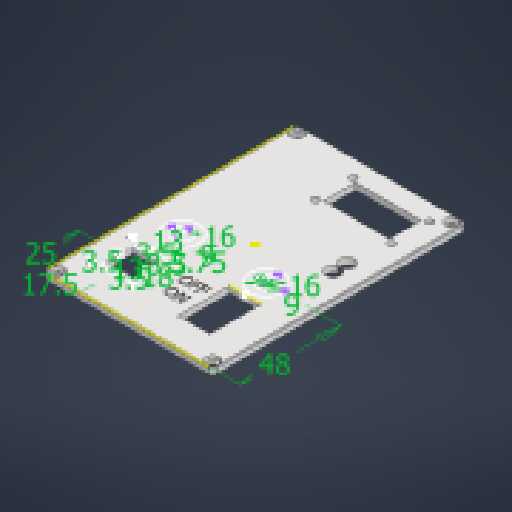
# Autodesk Inventor part: PCB_Housing_06_V4
Saved by Autodesk Inventor 2026.2 (Build 302298000, 298)
## iProperties
Created: 2026-03-17
Part Number: PCB_Housing_06_V4
Material: Generic
Document SubType Name: Modeling
Designer: vckot
Density: 1 g/cm^3
Appearance: Default
Author: vckot
Autodesk Inventor part; units mm, degrees
ref_plane "YZ Plane" through (0, 0, 0) normal (1, 0, 0) x (0, 1, 0)
ref_plane "XZ Plane" through (0, 0, 0) normal (0, 1, 0) x (-1, 0, 0)
ref_plane "XY Plane" through (0, 0, 0) normal (0, 0, 1) x (1, 0, 0)
sketch "Sketch1" plane through (0, 0, 0) normal (0, 1, 0) x (-1, 0, 0)
  line L0 (-40, 60) -> (40, 60)
  line L1 (40, 60) -> (40, -60)
  line L2 (40, -60) -> (-40, -60)
  line L3 (-40, -60) -> (-40, 60)
  line L4 (-40, 60) -> (40, -60) construction
  line L5 (40, 60) -> (-40, -60) construction
  point P0 (0, 0)
  dimension "d0" = 120
  dimension "d1" = 80
  constraints: 12 end point, 2 midpoint, 2 parallel, 1 horizontal, 1 perpendicular
  measures "d0" distance of L0.end L1.end
  measures "d1" distance of L0.start L0.end
extrude "Extrusion1" add sketch "Sketch1" along normal blind 3
sketch "Sketch2" plane through (0, 3, 0) normal (0, 1, 0) x (1, 0, 0)
  circle A0 centre (36.5, -56.5) radius 2.25 projected
  circle A1 centre (-36.5, 56.5) radius 2.25 projected
  circle A2 centre (36.5, 56.5) radius 2.25
  circle A3 centre (-36.5, -56.5) radius 2.25
  point P0 (0, 0)
  constraints: 2 centre point, 2 equal radius, 2 horizontal alignment, 2 vertical alignment
hole "Hole1" at (36.5, 3, 56.5) at (-36.5, 3, -56.5) at (36.5, 3, -56.5) at (-36.5, 3, 56.5) direction (0, -1, 0) diameter 3.75 depth 8 tip angle 118 counterbore diameter 6 counterbore depth 2
sketch "Sketch3" plane through (0, 3, 0) normal (0, 1, 0) x (1, 0, 0)
  line L0 (24.241, -45.543499) -> (24.241, -22.556499)
  line L1 (10.779, -45.543499) -> (24.241, -45.543499)
  line L2 (10.779, -22.556499) -> (10.779, -45.543499)
  line L3 (10.779, -22.556499) -> (24.241, -22.556499)
  arc A0 (26.856832, 17.449996) -> (30.143167, 17.449996) centre (28.499999, 14.999996) ccw
  arc A1 (26.856832, 10.949996) -> (30.143167, 10.949996) centre (28.499999, 8.499996) ccw
  circle A2 centre (28.499999, 8.499996) radius 2.95
  circle A3 centre (28.499999, 14.999996) radius 2.95
  line L4 (28, 35.5) -> (-2, 35.5)
  line L5 (-2, 35.5) -> (-2, 49.5)
  line L6 (-2, 49.5) -> (28, 49.5)
  line L7 (28, 49.5) -> (28, 35.5)
  circle A4 centre (-7, 34) radius 1.1
  circle A5 centre (30, 34) radius 1.1
  circle A6 centre (30, 52) radius 1.1
  circle A7 centre (-7, 52) radius 1.1
  line L8 (31.5, 32.5) -> (31.5, 53.5)
  line L9 (31.5, 53.5) -> (-8.5, 53.5)
  line L10 (-8.5, 53.5) -> (-8.5, 32.5)
  line L11 (-8.5, 32.5) -> (31.5, 32.5)
  point P0 (0, 0)
  point P1 (26.856832, 10.949996)
  constraints: 2 centre point, 2 coincident, 2 concentric, 2 end point, 1 horizontal
extrude "Extrusion2" cut sketch "Sketch3" against normal through all contours L1 L2 L3 L0 | A3 A0 | A2 A1 | L4 L5 L6 L7
sketch "Sketch5" plane through (0, 3, 0) normal (0, 1, 0) x (1, 0, 0)
  circle A0 centre (-5, 33.5) radius 1.75
  circle A1 centre (-5, 51.5) radius 1.75
  circle A2 centre (31, 51.5) radius 1.75
  circle A3 centre (31, 33.5) radius 1.75
  line L0 (28, 35.5) -> (-2, 35.5) projected
  line L1 (-2, 35.5) -> (-2, 49.5) projected
  line L2 (-2, 49.5) -> (28, 49.5) projected
  line L3 (28, 49.5) -> (28, 35.5) projected
  point P0 (0, 0)
  dimension "d27" = 3.5
  dimension "d28" = 2
  dimension "d29" = 3
  dimension "d30" = 2
  dimension "d31" = 3
  dimension "d32" = 3
  dimension "d33" = 3
  dimension "d34" = 2
  dimension "d35" = 2
  constraints: 4 centre point, 3 equal radius
  measures "d27" diameter of A0
  measures "d28" distance from line of A0.centre L0
  measures "d29" distance from line of L1 A0.centre
  measures "d30" distance from line of L2 A1.centre
  measures "d31" distance from line of L1 A1.centre
  measures "d32" distance from line of L3 A2.centre
  measures "d33" distance from line of L3 A3.centre
  measures "d34" distance from line of L0 A3.centre
  measures "d35" distance from line of L2 A2.centre
extrude "Extrusion4" cut sketch "Sketch5" against normal through all contours A0 | A1 | A2 | A3
thicken "Thicken1" operation add thickness 0.5 both sides no extend neighbours yes toward (0, 0, -1) faces at (18, 2, -49.5) (-2, 2, -44.833333) (28, 2, -40.166667) (8, 2, -35.5)
thicken "Thicken2" operation add thickness 0.5 both sides no extend neighbours yes toward (0.6830158, 0, -0.7304036) faces at (30.514896, 2, -17.154687)
thicken "Thicken3" operation add thickness 0.5 both sides no extend neighbours yes toward (0.6830158, 0, -0.7304036) faces at (30.514896, 2, -10.654687)
thicken "Thicken4" operation add thickness 0.75 both sides no extend neighbours yes toward (1, 0, 0) faces at (24.241, 1, 30.218832) (19.753666, 2, 22.556499) (10.779, 2, 30.218832) (15.266333, 2, 45.543499)
sketch "Sketch4" plane through (0, 3, 0) normal (0, 1, 0) x (1, 0, 0)
  line L0 (-9.166236, -22.743083) -> (11.364424, -22.743083) construction
  line L1 (11.364424, -22.743083) -> (11.364424, -45.356916) construction
  line L2 (11.364424, -45.356916) -> (-9.166236, -45.356916) construction
  line L3 (-9.166236, -45.356916) -> (-9.166236, -22.743083) construction
  line L4 (10.029, -21.806499) -> (24.991, -21.806499)
  line L5 (10.029, -46.293499) -> (10.029, -21.806499)
  spline S0 degree 2 poles (-0.87619, -28.005128) (-0.59256, -28.337381) (-0.276514, -29.309828) (-0.276514, -29.933815) knots 0 0 0 1 2 2 2
  spline S1 degree 2 poles (-0.276514, -29.933815) (-0.276514, -30.541595) (-0.584456, -31.526197) (-0.87619, -31.85845) knots 0 0 0 1 2 2 2
  spline S2 degree 2 poles (-0.87619, -31.85845) (-1.184132, -32.206911) (-1.998556, -32.539163) (-2.488832, -32.539163) knots 0 0 0 1 2 2 2
  spline S3 degree 2 poles (-2.488832, -32.539163) (-2.995315, -32.539163) (-3.805688, -32.194755) (-4.101474, -31.85845) knots 0 0 0 1 2 2 2
  spline S4 degree 2 poles (-4.101474, -31.85845) (-4.389156, -31.526197) (-4.697098, -30.549698) (-4.697098, -29.933815) knots 0 0 0 1 2 2 2
  spline S5 degree 2 poles (-4.697098, -29.933815) (-4.697098, -29.305776) (-4.385104, -28.349536) (-4.097422, -28.005128) knots 0 0 0 1 2 2 2
  spline S6 degree 2 poles (-4.097422, -28.005128) (-3.805688, -27.672875) (-2.991263, -27.328467) (-2.488832, -27.328467) knots 0 0 0 1 2 2 2
  spline S7 degree 2 poles (-2.488832, -27.328467) (-1.978297, -27.328467) (-1.159821, -27.685031) (-0.87619, -28.005128) knots 0 0 0 1 2 2 2
  spline S8 degree 2 poles (-0.969383, -29.933815) (-0.969383, -29.439488) (-1.184132, -28.673685) (-1.378621, -28.42247) knots 0 0 0 1 2 2 2
  spline S9 degree 2 poles (-1.378621, -28.42247) (-1.577162, -28.16315) (-2.13632, -27.903831) (-2.48478, -27.903831) knots 0 0 0 1 2 2 2
  spline S10 degree 2 poles (-2.48478, -27.903831) (-2.845396, -27.903831) (-3.388346, -28.155047) (-3.594991, -28.42247) knots 0 0 0 1 2 2 2
  spline S11 degree 2 poles (-3.594991, -28.42247) (-3.793532, -28.677737) (-4.004229, -29.447591) (-4.004229, -29.933815) knots 0 0 0 1 2 2 2
  spline S12 degree 2 poles (-4.004229, -29.933815) (-4.004229, -30.918418) (-3.177649, -31.963799) (-2.48478, -31.963799) knots 0 0 0 1 2 2 2
  spline S13 degree 2 poles (-2.48478, -31.963799) (-1.791911, -31.963799) (-0.969383, -30.918418) (-0.969383, -29.933815) knots 0 0 0 1 2 2 2
  line L6 (3.443097, -28.025387) -> (1.117327, -28.025387)
  line L7 (1.117327, -28.025387) -> (1.117327, -29.435436)
  line L8 (1.117327, -29.435436) -> (3.345852, -29.435436)
  line L9 (3.345852, -29.435436) -> (3.345852, -30.027008)
  line L10 (3.345852, -30.027008) -> (1.117327, -30.027008)
  line L11 (1.117327, -30.027008) -> (1.117327, -32.433815)
  line L12 (1.117327, -32.433815) -> (0.452821, -32.433815)
  line L13 (0.452821, -32.433815) -> (0.452821, -27.433815)
  line L14 (0.452821, -27.433815) -> (3.443097, -27.433815)
  line L15 (3.443097, -27.433815) -> (3.443097, -28.025387)
  line L16 (7.028996, -28.025387) -> (4.703226, -28.025387)
  line L17 (4.703226, -28.025387) -> (4.703226, -29.435436)
  line L18 (4.703226, -29.435436) -> (6.931752, -29.435436)
  line L19 (6.931752, -29.435436) -> (6.931752, -30.027008)
  line L20 (6.931752, -30.027008) -> (4.703226, -30.027008)
  line L21 (4.703226, -30.027008) -> (4.703226, -32.433815)
  line L22 (4.703226, -32.433815) -> (4.038721, -32.433815)
  line L23 (4.038721, -32.433815) -> (4.038721, -27.433815)
  line L24 (4.038721, -27.433815) -> (7.028996, -27.433815)
  line L25 (7.028996, -27.433815) -> (7.028996, -28.025387)
  spline S14 degree 2 poles (0.414329, -36.237496) (0.697959, -36.569749) (1.014005, -37.542196) (1.014005, -38.166183) knots 0 0 0 1 2 2 2
  spline S15 degree 2 poles (1.014005, -38.166183) (1.014005, -38.773963) (0.706063, -39.758566) (0.414329, -40.090819) knots 0 0 0 1 2 2 2
  spline S16 degree 2 poles (0.414329, -40.090819) (0.106387, -40.439279) (-0.708037, -40.771532) (-1.198313, -40.771532) knots 0 0 0 1 2 2 2
  spline S17 degree 2 poles (-1.198313, -40.771532) (-1.704796, -40.771532) (-2.515169, -40.427123) (-2.810955, -40.090819) knots 0 0 0 1 2 2 2
  spline S18 degree 2 poles (-2.810955, -40.090819) (-3.098637, -39.758566) (-3.406579, -38.782067) (-3.406579, -38.166183) knots 0 0 0 1 2 2 2
  spline S19 degree 2 poles (-3.406579, -38.166183) (-3.406579, -37.538144) (-3.094585, -36.581904) (-2.806903, -36.237496) knots 0 0 0 1 2 2 2
  spline S20 degree 2 poles (-2.806903, -36.237496) (-2.515169, -35.905243) (-1.700744, -35.560835) (-1.198313, -35.560835) knots 0 0 0 1 2 2 2
  spline S21 degree 2 poles (-1.198313, -35.560835) (-0.687778, -35.560835) (0.130698, -35.917399) (0.414329, -36.237496) knots 0 0 0 1 2 2 2
  spline S22 degree 2 poles (0.321136, -38.166183) (0.321136, -37.671856) (0.106387, -36.906054) (-0.088102, -36.654838) knots 0 0 0 1 2 2 2
  spline S23 degree 2 poles (-0.088102, -36.654838) (-0.286644, -36.395519) (-0.845801, -36.136199) (-1.194261, -36.136199) knots 0 0 0 1 2 2 2
  spline S24 degree 2 poles (-1.194261, -36.136199) (-1.554877, -36.136199) (-2.097827, -36.387415) (-2.304472, -36.654838) knots 0 0 0 1 2 2 2
  spline S25 degree 2 poles (-2.304472, -36.654838) (-2.503013, -36.910105) (-2.71371, -37.67996) (-2.71371, -38.166183) knots 0 0 0 1 2 2 2
  spline S26 degree 2 poles (-2.71371, -38.166183) (-2.71371, -39.150786) (-1.88713, -40.196167) (-1.194261, -40.196167) knots 0 0 0 1 2 2 2
  spline S27 degree 2 poles (-1.194261, -40.196167) (-0.501392, -40.196167) (0.321136, -39.150786) (0.321136, -38.166183) knots 0 0 0 1 2 2 2
  line L26 (5.321136, -40.666183) -> (4.575593, -40.666183)
  line L27 (4.575593, -40.666183) -> (2.363275, -36.355)
  line L28 (2.363275, -36.355) -> (2.363275, -40.666183)
  line L29 (2.363275, -40.666183) -> (1.74334, -40.666183)
  line L30 (1.74334, -40.666183) -> (1.74334, -35.666183)
  line L31 (1.74334, -35.666183) -> (2.687425, -35.666183)
  line L32 (2.687425, -35.666183) -> (4.701201, -39.624854)
  line L33 (4.701201, -39.624854) -> (4.701201, -35.666183)
  line L34 (4.701201, -35.666183) -> (5.321136, -35.666183)
  line L35 (5.321136, -35.666183) -> (5.321136, -40.666183)
  point P0 (0, 0)
  point P1 (11.364424, -34.049999)
  point P2 (10.029, -34.049999)
  dimension "d0" = 120
  dimension "d1" = 80
  constraints: 2 midpoint, 1 horizontal alignment, 2 other
extrude "Extrusion3" cut sketch "Sketch4" against normal blind 2
fillet "Fillet1" radius 2 4 edges at (-40, 1.5, -60) (-40, 1.5, 60) (40, 1.5, -60) (40, 1.5, 60)
fillet "Fillet2" radius 0.5 8 edges at (39.4142, 3, -59.4142) (0, 3, -60) (-39.4142, 3, -59.4142) (-40, 3, 0) (-39.4142, 3, 59.4142) (0, 3, 60) (39.4142, 3, 59.4142) (40, 3, 0)
sketch "Sketch6" plane through (0, 3, 0) normal (0, 1, 0) x (1, 0, 0)
  line L0 (8.988356, -6.885061) -> (26.031643, -6.885061) construction
  line L1 (26.031643, -6.885061) -> (26.031643, -17.114939) construction
  line L2 (26.031643, -17.114939) -> (8.988356, -17.114939) construction
  line L3 (8.988356, -17.114939) -> (8.988356, -6.885061) construction
  circle A0 centre (17.51, -12) radius 4.5
  circle A1 centre (17.51, -12) radius 8
  line L4 (10.029, -21.806499) -> (24.991, -21.806499)
  line L5 (-26.5, -31) -> (-13.5, -31)
  line L6 (-13.5, -31) -> (-13.5, -49)
  line L7 (-13.5, -49) -> (-26.5, -49)
  line L8 (-26.5, -49) -> (-26.5, -31)
  line L9 (-40, 58) -> (-40, -58)
  line L10 (-38, -60) -> (38, -60)
  line L11 (-26.5, -33.5) -> (-13.5, -33.5)
  line L12 (-13.5, -33.5) -> (-13.5, -46.5)
  line L13 (-13.5, -46.5) -> (-26.5, -46.5)
  line L14 (-26.5, -46.5) -> (-26.5, -33.5)
  circle A2 centre (-20, -12) radius 4.5
  circle A3 centre (-20, -12) radius 8
  line L15 (-27.288736, -8.885737) -> (-12.711264, -8.885737) construction
  line L16 (-12.711264, -8.885737) -> (-12.711264, -15.114263) construction
  line L17 (-12.711264, -15.114263) -> (-27.288736, -15.114263) construction
  line L18 (-27.288736, -15.114263) -> (-27.288736, -8.885737) construction
  circle A4 centre (-10, -30) radius 1.875
  circle A5 centre (-30, -30) radius 1.875
  circle A6 centre (-30, -50) radius 1.875
  circle A7 centre (-10, -50) radius 1.875
  point P0 (0, 0)
  point P1 (17.51, -21.806499)
  point P2 (-20, -49)
  point P3 (-13.5, -40)
  point P4 (-26.5, -40)
  point P5 (-26.5, -40)
  point P6 (-20, -31)
  point P7 (-20, -8.885737)
  point P8 (-27.288736, -12)
  point P9 (26.031643, -12)
  point P10 (17.51, -6.885061)
  point P11 (-26.5, -46.5)
  point P12 (-13.5, -33.5)
  dimension "d0" = 120
  dimension "d1" = 80
  dimension "d38" = 16
  dimension "d39" = 9
  dimension "d40" = 18
  dimension "d41" = 13
  dimension "d42" = 20
  dimension "d43" = 20
  dimension "d44" = 13
  dimension "d45" = 48
  dimension "d46" = 16
  dimension "d47" = 9
  dimension "d48" = 3.75
  dimension "d50" = 3.5
  dimension "d51" = 3.5
  dimension "d52" = 3.5
  dimension "d53" = 3.5
  constraints: 16 end point, 10 midpoint, 8 centre point, 6 vertical alignment, 5 horizontal alignment, 4 parallel, 3 coincident, 3 equal radius, 2 horizontal, 2 perpendicular, 2 point on line, 4 other
  measures "d38" diameter of A1
  measures "d39" diameter of A0
  measures "d40" distance between parallel lines of L7 L5
  measures "d41" distance between parallel lines of L8 L6
  measures "d42" distance from line of L9 point (-20, -49)
  measures "d43" distance from line of L10 point (-13.5, -40)
  measures "d44" distance between parallel lines of L13 L11
  measures "d45" distance from line of L10 A1.centre
  measures "d46" diameter of A3
  measures "d47" diameter of A2
  measures "d48" diameter of A4
  measures "d50" distance from line of A4.centre L11
  measures "d51" distance from line of A4.centre L12
  measures "d52" distance from line of L13 A7.centre
  measures "d53" distance from line of A6.centre L8
extrude "Extrusion5" cut sketch "Sketch6" against normal blind 2.5 contours L11 L6 L13 L8
extrude "Extrusion7" cut sketch "Sketch6" against normal blind 10 contours L11 L6 L13 L8 | A4 | A5 | A6 | A7
body "Solid1"
